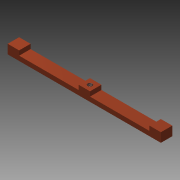
# Autodesk Inventor part: top_conductor
Saved by Autodesk Inventor 2014 SP1 (Build 180222100, 222)
## iProperties
Created: 2016-08-31
Part Number: top_conductor
Material: Copper, Alloy
Document SubType Name: Modeling
Designer: tguillod
Density: 7.58 g/cm^3
Appearance: Copper - Satin
Author: tguillod
Autodesk Inventor part; units mm, degrees
ref_plane "YZ Plane" through (0, 0, 0) normal (1, 0, 0) x (0, 1, 0)
ref_plane "XZ Plane" through (0, 0, 0) normal (0, 1, 0) x (-1, 0, 0)
ref_plane "XY Plane" through (0, 0, 0) normal (0, 0, 1) x (1, 0, 0)
sketch "Sketch1" plane through (0, 0, 0) normal (0, 0, 1) x (1, 0, 0)
  line L0 (0, 0) -> (67, 0)
  line L1 (67, 0) -> (67, 5)
  line L2 (67, 5) -> (0, 5)
  line L3 (0, 5) -> (0, 0)
  dimension "d0" = 5
  dimension "d1" = 67
  constraints: 8 end point, 2 parallel, 1 horizontal, 1 perpendicular
  measures "d0" distance of L0.end L1.end
  measures "d1" distance of L1.end L2.end
extrude "Extrusion1" add sketch "Sketch1" along normal blind 2
sketch "Sketch2" plane through (0, 0, 2) normal (0, 0, 1) x (1, 0, 0)
  line L0 (0, 0) -> (67, 0) projected
  line L1 (67, 0) -> (67, 5) projected
  line L2 (67, 5) -> (0, 5) projected
  line L3 (0, 5) -> (0, 0) projected
  line L4 (0, 5) -> (5, 5)
  line L5 (5, 5) -> (5, 0)
  line L6 (5, 0) -> (0, 0)
  line L7 (0, 0) -> (0, 5)
  line L8 (31, 5) -> (36, 5)
  line L9 (36, 5) -> (36, 0)
  line L10 (36, 0) -> (31, 0)
  line L11 (31, 0) -> (31, 5)
  line L12 (67, 5) -> (62, 5)
  line L13 (62, 5) -> (62, 0)
  line L14 (62, 0) -> (67, 0)
  line L15 (67, 0) -> (67, 5)
  dimension "d4" = 5
  dimension "d5" = 5
  dimension "d7" = 26
  dimension "d8" = 26
  constraints: 24 end point, 6 parallel, 4 point on line, 3 horizontal, 3 perpendicular
  measures "d4" distance between parallel lines of L3 L5
  measures "d5" distance between parallel lines of L1 L13
  measures "d7" distance between parallel lines of L11 L5
  measures "d8" distance between parallel lines of L13 L9
extrude "Extrusion2" add sketch "Sketch2" along normal blind 2 contours L3 L2 L5 L0 | L11 L2 L9 L0 | L13 L2 L1 L0
sketch "Sketch4" plane through (0, 0, 0) normal (0, 0, -1) x (-1, 0, 0)
  line L0 (0, 0) -> (-67, 0) projected
  line L1 (0, 5) -> (0, 0) projected
  line L2 (-67, 5) -> (0, 5) projected
  line L3 (-67, 0) -> (-67, 5) projected
  line L4 (-67, 2.5) -> (0, 2.5) construction
  line L5 (-33.5, 5) -> (-33.5, 0) construction
  point P0 (-33.5, 2.5)
  constraints: 6 midpoint, 4 end point
hole "Hole1" at (33.5, 2.5, 0) direction (0, 0, 1) diameter 2.013 end through all thread size "M2.5x0.45" class "6H" standard "ISO Metric profile"
body "Solid1"
